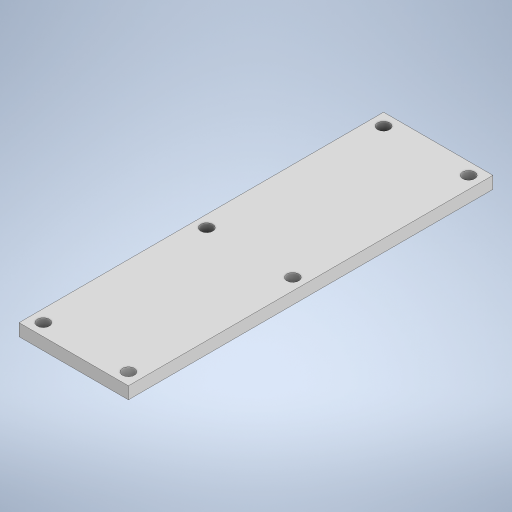
# Autodesk Inventor part: BaseM
Saved by Autodesk Inventor 2024 (Build 280153020, 153B)
## iProperties
Created: 2023-06-05
Part Number: BaseM
Material: Genérico
Document SubType Name: Modeling
Designer: victo
Density: 1 g/cm^3
Appearance: Padrão
Author: victo
Autodesk Inventor part; units mm, degrees
ref_plane "YZ Plane" through (0, 0, 0) normal (1, 0, 0) x (0, 1, 0)
ref_plane "XZ Plane" through (0, 0, 0) normal (0, 1, 0) x (-1, 0, 0)
ref_plane "XY Plane" through (0, 0, 0) normal (0, 0, 1) x (1, 0, 0)
sketch "Esboço1" plane through (0, 0, 0) normal (0, 1, 0) x (-1, 0, 0)
  line L0 (0, 0) -> (0, 150)
  line L1 (0, 150) -> (45, 150)
  line L2 (45, 150) -> (45, 0)
  line L3 (45, 0) -> (0, 0)
  line L4 (45, 0) -> (55, 0)
  circle A0 centre (5, 5) radius 2.5
  circle A1 centre (5, 145) radius 2.5
  circle A2 centre (40, 145) radius 2.5
  circle A3 centre (40, 5) radius 2.5
  circle A4 centre (40.2, 77.5645) radius 2.5
  circle A5 centre (4.8, 77.5645) radius 2.5
  dimension "d0" = 150
  dimension "d1" = 45
  dimension "d10" = 5
  dimension "d12" = 5
  dimension "d22" = 5
  dimension "d23" = 5
  dimension "d29" = 5
  dimension "d30" = 5
  constraints: 10 end point, 6 centre point, 3 perpendicular, 1 horizontal, 1 vertical
  measures "d0" distance of L0.start L0.end
  measures "d1" distance of L0.end L1.end
  measures "d10" diameter of A0
  measures "d12" diameter of A1
  measures "d22" diameter of A2
  measures "d23" diameter of A3
  measures "d29" diameter of A4
  measures "d30" diameter of A5
extrude "Extrusão5" add sketch "Esboço1" along normal blind 5
